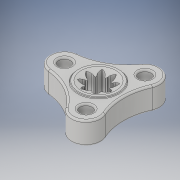
# Autodesk Inventor part: gear sleeve
Saved by Autodesk Inventor 2017 (Build 210142000, 142)
## iProperties
Created: 2020-09-28
Part Number: gear sleeve
Material: Generic
Document SubType Name: Modeling
Designer: Brandt
Density: 1 g/cm^3
Appearance: Default
Author: Brandt
Autodesk Inventor part; units mm, degrees
ref_plane "YZ Plane" through (0, 0, 0) normal (1, 0, 0) x (0, 1, 0)
ref_plane "XZ Plane" through (0, 0, 0) normal (0, 1, 0) x (-1, 0, 0)
ref_plane "XY Plane" through (0, 0, 0) normal (0, 0, 1) x (1, 0, 0)
sketch "Sketch10" plane through (0, 0, 0) normal (0, 1, 0) x (-1, 0, 0)
  circle A0 centre (0, 0) radius 10.9855
  dimension "d120" = 21.971
  constraints: 1 centre point, 1 coincident
  measures "d120" diameter of A0
extrude "Extrusion9" add sketch "Sketch10" along normal blind 5.461
sketch "Sketch12" plane through (0, 0, 0) normal (0, -1, 0) x (-1, 0, 0)
  arc A0 (-1.0187, 1.6285) -> (-1.0516, 1.6075) centre (0, 0) ccw construction
  arc A1 (-1.4637, 1.6634) -> (-1.0516, 1.6075) centre (-1.2254, 1.8732) ccw construction
  line L0 (-1.4637, 1.6634) -> (-1.4758, 1.6771) construction
  arc A2 (-1.4758, 1.6771) -> (-1.5461, 1.7343) centre (-1.6809, 1.4966) ccw construction
  arc A3 (-1.5461, 1.7343) -> (-1.876, 1.8563) centre (-2.085, 0.7843) ccw construction
  arc A4 (-1.876, 1.8563) -> (-2.5953, 1.8563) centre (-2.2357, 0.0114) ccw construction
  arc A5 (-2.5953, 1.8563) -> (-2.6389, 1.7938) centre (0, 0) ccw construction
  arc A6 (-2.6389, 1.7938) -> (-2.3903, 1.1188) centre (-0.7834, 2.0939) ccw construction
  arc A7 (-2.3903, 1.1188) -> (-2.1618, 0.8514) centre (-1.4566, 1.6854) ccw construction
  arc A8 (-2.1618, 0.8514) -> (-2.0838, 0.8052) centre (-1.9853, 1.0601) ccw construction
  line L1 (-2.0838, 0.8052) -> (-2.0668, 0.7986) construction
  arc A9 (-1.8719, 0.4312) -> (-2.0668, 0.7986) centre (-2.1813, 0.5024) ccw construction
  arc A10 (-1.8719, 0.4312) -> (-1.8802, 0.3931) centre (0, 0) ccw construction
  arc A11 (-2.2112, 0.1412) -> (-1.8802, 0.3931) centre (-2.191, 0.4581) ccw construction
  line L2 (-2.2112, 0.1412) -> (-2.2294, 0.1424) construction
  arc A12 (-2.2294, 0.1424) -> (-2.3196, 0.1331) centre (-2.2468, -0.1304) ccw construction
  arc A13 (-2.3196, 0.1331) -> (-2.6391, -0.0139) centre (-2.0289, -0.9197) ccw construction
  arc A14 (-2.6391, -0.0139) -> (-3.1478, -0.5226) centre (-1.5889, -1.5728) ccw construction
  arc A15 (-3.1478, -0.5226) -> (-3.1344, -0.5976) centre (0, 0) ccw construction
  arc A16 (-3.1344, -0.5976) -> (-2.4813, -0.8991) centre (-2.0346, 0.9266) ccw construction
  arc A17 (-2.4813, -0.8991) -> (-2.1306, -0.9266) centre (-2.2217, 0.1618) ccw construction
  arc A18 (-2.1306, -0.9266) -> (-2.0428, -0.9042) centre (-2.1534, -0.6542) ccw construction
  line L3 (-2.0428, -0.9042) -> (-2.0262, -0.8968) construction
  arc A19 (-1.6285, -1.0187) -> (-2.0262, -0.8968) centre (-1.8977, -1.1871) ccw construction
  arc A20 (-1.6285, -1.0187) -> (-1.6075, -1.0516) centre (0, 0) ccw construction
  arc A21 (-1.6634, -1.4637) -> (-1.6075, -1.0516) centre (-1.8732, -1.2254) ccw construction
  line L4 (-1.6634, -1.4637) -> (-1.6771, -1.4758) construction
  arc A22 (-1.6771, -1.4758) -> (-1.7343, -1.5461) centre (-1.4966, -1.6809) ccw construction
  arc A23 (-1.7343, -1.5461) -> (-1.8563, -1.876) centre (-0.7843, -2.085) ccw construction
  arc A24 (-1.8563, -1.876) -> (-1.8563, -2.5953) centre (-0.0114, -2.2357) ccw construction
  arc A25 (-1.8563, -2.5953) -> (-1.7938, -2.6389) centre (0, 0) ccw construction
  arc A26 (-1.7938, -2.6389) -> (-1.1188, -2.3903) centre (-2.0939, -0.7834) ccw construction
  arc A27 (-1.1188, -2.3903) -> (-0.8514, -2.1618) centre (-1.6854, -1.4566) ccw construction
  arc A28 (-0.8514, -2.1618) -> (-0.8052, -2.0838) centre (-1.0601, -1.9853) ccw construction
  line L5 (-0.8052, -2.0838) -> (-0.7986, -2.0668) construction
  arc A29 (-0.4312, -1.8719) -> (-0.7986, -2.0668) centre (-0.5024, -2.1813) ccw construction
  arc A30 (-0.4312, -1.8719) -> (-0.3931, -1.8802) centre (0, 0) ccw construction
  arc A31 (-0.1412, -2.2112) -> (-0.3931, -1.8802) centre (-0.4581, -2.191) ccw construction
  line L6 (-0.1412, -2.2112) -> (-0.1424, -2.2294) construction
  arc A32 (-0.1424, -2.2294) -> (-0.1331, -2.3196) centre (0.1304, -2.2468) ccw construction
  arc A33 (-0.1331, -2.3196) -> (0.0139, -2.6391) centre (0.9197, -2.0289) ccw construction
  arc A34 (0.0139, -2.6391) -> (0.5226, -3.1478) centre (1.5728, -1.5889) ccw construction
  arc A35 (0.5226, -3.1478) -> (0.5976, -3.1344) centre (0, 0) ccw construction
  arc A36 (0.5976, -3.1344) -> (0.8991, -2.4813) centre (-0.9266, -2.0346) ccw construction
  arc A37 (0.8991, -2.4813) -> (0.9266, -2.1306) centre (-0.1618, -2.2217) ccw construction
  arc A38 (0.9266, -2.1306) -> (0.9042, -2.0428) centre (0.6542, -2.1534) ccw construction
  line L7 (0.9042, -2.0428) -> (0.8968, -2.0262) construction
  arc A39 (1.0187, -1.6285) -> (0.8968, -2.0262) centre (1.1871, -1.8977) ccw construction
  arc A40 (1.0187, -1.6285) -> (1.0516, -1.6075) centre (0, 0) ccw construction
  arc A41 (1.4637, -1.6634) -> (1.0516, -1.6075) centre (1.2254, -1.8732) ccw construction
  line L8 (1.4637, -1.6634) -> (1.4758, -1.6771) construction
  arc A42 (1.4758, -1.6771) -> (1.5461, -1.7343) centre (1.6809, -1.4966) ccw construction
  arc A43 (1.5461, -1.7343) -> (1.876, -1.8563) centre (2.085, -0.7843) ccw construction
  arc A44 (1.876, -1.8563) -> (2.5953, -1.8563) centre (2.2357, -0.0114) ccw construction
  arc A45 (2.5953, -1.8563) -> (2.6389, -1.7938) centre (0, 0) ccw construction
  arc A46 (2.6389, -1.7938) -> (2.3903, -1.1188) centre (0.7834, -2.0939) ccw construction
  arc A47 (2.3903, -1.1188) -> (2.1618, -0.8514) centre (1.4566, -1.6854) ccw construction
  arc A48 (2.1618, -0.8514) -> (2.0838, -0.8052) centre (1.9853, -1.0601) ccw construction
  line L9 (2.0838, -0.8052) -> (2.0668, -0.7986) construction
  arc A49 (1.8719, -0.4312) -> (2.0668, -0.7986) centre (2.1813, -0.5024) ccw construction
  arc A50 (1.8719, -0.4312) -> (1.8802, -0.3931) centre (0, 0) ccw construction
  arc A51 (2.2112, -0.1412) -> (1.8802, -0.3931) centre (2.191, -0.4581) ccw construction
  line L10 (2.2112, -0.1412) -> (2.2294, -0.1424) construction
  arc A52 (2.2294, -0.1424) -> (2.3196, -0.1331) centre (2.2468, 0.1304) ccw construction
  arc A53 (2.3196, -0.1331) -> (2.6391, 0.0139) centre (2.0289, 0.9197) ccw construction
  arc A54 (2.6391, 0.0139) -> (3.1478, 0.5226) centre (1.5889, 1.5728) ccw construction
  arc A55 (3.1478, 0.5226) -> (3.1344, 0.5976) centre (0, 0) ccw construction
  arc A56 (3.1344, 0.5976) -> (2.4813, 0.8991) centre (2.0346, -0.9266) ccw construction
  arc A57 (2.4813, 0.8991) -> (2.1306, 0.9266) centre (2.2217, -0.1618) ccw construction
  arc A58 (2.1306, 0.9266) -> (2.0428, 0.9042) centre (2.1534, 0.6542) ccw construction
  line L11 (2.0428, 0.9042) -> (2.0262, 0.8968) construction
  arc A59 (1.6285, 1.0187) -> (2.0262, 0.8968) centre (1.8977, 1.1871) ccw construction
  arc A60 (1.6285, 1.0187) -> (1.6075, 1.0516) centre (0, 0) ccw construction
  arc A61 (1.6634, 1.4637) -> (1.6075, 1.0516) centre (1.8732, 1.2254) ccw construction
  line L12 (1.6634, 1.4637) -> (1.6771, 1.4758) construction
  arc A62 (1.6771, 1.4758) -> (1.7343, 1.5461) centre (1.4966, 1.6809) ccw construction
  arc A63 (1.7343, 1.5461) -> (1.8563, 1.876) centre (0.7843, 2.085) ccw construction
  arc A64 (1.8563, 1.876) -> (1.8563, 2.5953) centre (0.0114, 2.2357) ccw construction
  arc A65 (1.8563, 2.5953) -> (1.7938, 2.6389) centre (0, 0) ccw construction
  arc A66 (1.7938, 2.6389) -> (1.1188, 2.3903) centre (2.0939, 0.7834) ccw construction
  arc A67 (1.1188, 2.3903) -> (0.8514, 2.1618) centre (1.6854, 1.4566) ccw construction
  arc A68 (0.8514, 2.1618) -> (0.8052, 2.0838) centre (1.0601, 1.9853) ccw construction
  line L13 (0.8052, 2.0838) -> (0.7986, 2.0668) construction
  arc A69 (0.4312, 1.8719) -> (0.7986, 2.0668) centre (0.5024, 2.1813) ccw construction
  arc A70 (0.4312, 1.8719) -> (0.3931, 1.8802) centre (0, 0) ccw construction
  arc A71 (0.1412, 2.2112) -> (0.3931, 1.8802) centre (0.4581, 2.191) ccw construction
  line L14 (0.1412, 2.2112) -> (0.1424, 2.2294) construction
  arc A72 (0.1424, 2.2294) -> (0.1331, 2.3196) centre (-0.1304, 2.2468) ccw construction
  arc A73 (0.1331, 2.3196) -> (-0.0139, 2.6391) centre (-0.9197, 2.0289) ccw construction
  arc A74 (-0.0139, 2.6391) -> (-0.5226, 3.1478) centre (-1.5728, 1.5889) ccw construction
  arc A75 (-0.5226, 3.1478) -> (-0.5976, 3.1344) centre (0, 0) ccw construction
  arc A76 (-0.5976, 3.1344) -> (-0.8991, 2.4813) centre (0.9266, 2.0346) ccw construction
  arc A77 (-0.8991, 2.4813) -> (-0.9266, 2.1306) centre (0.1618, 2.2217) ccw construction
  arc A78 (-0.9266, 2.1306) -> (-0.9042, 2.0428) centre (-0.6542, 2.1534) ccw construction
  line L15 (-0.9042, 2.0428) -> (-0.8968, 2.0262) construction
  arc A79 (-1.0187, 1.6285) -> (-0.8968, 2.0262) centre (-1.1871, 1.8977) ccw construction
  circle A80 centre (0, 0) radius 8.0242 construction
  arc A81 (10.9855, 0) -> (10.9855, 0) centre (0, 0) ccw projected
  line L16 (-2.1126, 0.6801) -> (-2.1296, 0.6867)
  arc A82 (-2.2438, 0.7544) -> (-2.1296, 0.6867) centre (-1.9853, 1.0601) ccw
  arc A83 (-2.4989, 1.0529) -> (-2.2438, 0.7544) centre (-1.4566, 1.6854) ccw
  arc A84 (-2.7718, 1.8236) -> (-2.4989, 1.0529) centre (-0.7834, 2.0939) ccw
  arc A85 (-2.6693, 1.9706) -> (-2.7718, 1.8236) centre (0, 0) ccw
  arc A86 (-1.8517, 1.981) -> (-2.6693, 1.9706) centre (-2.2357, 0.0114) ccw
  arc A87 (-1.4834, 1.8448) -> (-1.8517, 1.981) centre (-2.085, 0.7843) ccw
  arc A88 (-1.3804, 1.761) -> (-1.4834, 1.8448) centre (-1.6809, 1.4966) ccw
  line L17 (-1.3804, 1.761) -> (-1.3684, 1.7473)
  arc A89 (-1.3684, 1.7473) -> (-1.1211, 1.7138) centre (-1.2254, 1.8732) ccw
  arc A90 (-1.0861, 1.7361) -> (-1.1211, 1.7138) centre (0, 0) ccw
  arc A91 (-1.0861, 1.7361) -> (-1.0129, 1.9748) centre (-1.1871, 1.8977) ccw
  line L18 (-1.0129, 1.9748) -> (-1.0203, 1.9914)
  arc A92 (-1.0532, 2.12) -> (-1.0203, 1.9914) centre (-0.6542, 2.1534) ccw
  arc A93 (-1.0225, 2.5115) -> (-1.0532, 2.12) centre (0.1618, 2.2217) ccw
  arc A94 (-0.6704, 3.2494) -> (-1.0225, 2.5115) centre (0.9266, 2.0346) ccw
  arc A95 (-0.494, 3.2809) -> (-0.6704, 3.2494) centre (0, 0) ccw
  arc A96 (0.0914, 2.7101) -> (-0.494, 3.2809) centre (-1.5728, 1.5889) ccw
  arc A97 (0.2555, 2.3534) -> (0.0914, 2.7101) centre (-0.9197, 2.0289) ccw
  arc A98 (0.2691, 2.2213) -> (0.2555, 2.3534) centre (-0.1304, 2.2468) ccw
  line L19 (0.2691, 2.2213) -> (0.268, 2.2031)
  arc A99 (0.268, 2.2031) -> (0.4191, 2.0045) centre (0.4581, 2.191) ccw
  arc A100 (0.4597, 1.9956) -> (0.4191, 2.0045) centre (0, 0) ccw
  arc A101 (0.4597, 1.9956) -> (0.6801, 2.1126) centre (0.5024, 2.1813) ccw
  line L20 (0.6801, 2.1126) -> (0.6867, 2.1296)
  arc A102 (0.7544, 2.2438) -> (0.6867, 2.1296) centre (1.0601, 1.9853) ccw
  arc A103 (1.0529, 2.4989) -> (0.7544, 2.2438) centre (1.6854, 1.4566) ccw
  arc A104 (1.8236, 2.7718) -> (1.0529, 2.4989) centre (2.0939, 0.7834) ccw
  arc A105 (1.9706, 2.6693) -> (1.8236, 2.7718) centre (0, 0) ccw
  arc A106 (1.981, 1.8517) -> (1.9706, 2.6693) centre (0.0114, 2.2357) ccw
  arc A107 (1.8448, 1.4834) -> (1.981, 1.8517) centre (0.7843, 2.085) ccw
  arc A108 (1.761, 1.3804) -> (1.8448, 1.4834) centre (1.4966, 1.6809) ccw
  line L21 (1.761, 1.3804) -> (1.7473, 1.3684)
  arc A109 (1.7473, 1.3684) -> (1.7138, 1.1211) centre (1.8732, 1.2254) ccw
  arc A110 (1.7361, 1.0861) -> (1.7138, 1.1211) centre (0, 0) ccw
  arc A111 (1.7361, 1.0861) -> (1.9748, 1.0129) centre (1.8977, 1.1871) ccw
  line L22 (1.9748, 1.0129) -> (1.9914, 1.0203)
  arc A112 (2.12, 1.0532) -> (1.9914, 1.0203) centre (2.1534, 0.6542) ccw
  arc A113 (2.5115, 1.0225) -> (2.12, 1.0532) centre (2.2217, -0.1618) ccw
  arc A114 (3.2494, 0.6704) -> (2.5115, 1.0225) centre (2.0346, -0.9266) ccw
  arc A115 (3.2809, 0.494) -> (3.2494, 0.6704) centre (0, 0) ccw
  arc A116 (2.7101, -0.0914) -> (3.2809, 0.494) centre (1.5889, 1.5728) ccw
  arc A117 (2.3534, -0.2555) -> (2.7101, -0.0914) centre (2.0289, 0.9197) ccw
  arc A118 (2.2213, -0.2691) -> (2.3534, -0.2555) centre (2.2468, 0.1304) ccw
  line L23 (2.2213, -0.2691) -> (2.2031, -0.268)
  arc A119 (2.2031, -0.268) -> (2.0045, -0.4191) centre (2.191, -0.4581) ccw
  arc A120 (1.9956, -0.4597) -> (2.0045, -0.4191) centre (0, 0) ccw
  arc A121 (1.9956, -0.4597) -> (2.1126, -0.6801) centre (2.1813, -0.5024) ccw
  line L24 (2.1126, -0.6801) -> (2.1296, -0.6867)
  arc A122 (2.2438, -0.7544) -> (2.1296, -0.6867) centre (1.9853, -1.0601) ccw
  arc A123 (2.4989, -1.0529) -> (2.2438, -0.7544) centre (1.4566, -1.6854) ccw
  arc A124 (2.7718, -1.8236) -> (2.4989, -1.0529) centre (0.7834, -2.0939) ccw
  arc A125 (2.6693, -1.9706) -> (2.7718, -1.8236) centre (0, 0) ccw
  arc A126 (1.8517, -1.981) -> (2.6693, -1.9706) centre (2.2357, -0.0114) ccw
  arc A127 (1.4834, -1.8448) -> (1.8517, -1.981) centre (2.085, -0.7843) ccw
  arc A128 (1.3804, -1.761) -> (1.4834, -1.8448) centre (1.6809, -1.4966) ccw
  line L25 (1.3804, -1.761) -> (1.3684, -1.7473)
  arc A129 (1.3684, -1.7473) -> (1.1211, -1.7138) centre (1.2254, -1.8732) ccw
  arc A130 (1.0861, -1.7361) -> (1.1211, -1.7138) centre (0, 0) ccw
  arc A131 (1.0861, -1.7361) -> (1.0129, -1.9748) centre (1.1871, -1.8977) ccw
  line L26 (1.0129, -1.9748) -> (1.0203, -1.9914)
  arc A132 (1.0532, -2.12) -> (1.0203, -1.9914) centre (0.6542, -2.1534) ccw
  arc A133 (1.0225, -2.5115) -> (1.0532, -2.12) centre (-0.1618, -2.2217) ccw
  arc A134 (0.6704, -3.2494) -> (1.0225, -2.5115) centre (-0.9266, -2.0346) ccw
  arc A135 (0.494, -3.2809) -> (0.6704, -3.2494) centre (0, 0) ccw
  arc A136 (-0.0914, -2.7101) -> (0.494, -3.2809) centre (1.5728, -1.5889) ccw
  arc A137 (-0.2555, -2.3534) -> (-0.0914, -2.7101) centre (0.9197, -2.0289) ccw
  arc A138 (-0.2691, -2.2213) -> (-0.2555, -2.3534) centre (0.1304, -2.2468) ccw
  line L27 (-0.2691, -2.2213) -> (-0.268, -2.2031)
  arc A139 (-0.268, -2.2031) -> (-0.4191, -2.0045) centre (-0.4581, -2.191) ccw
  arc A140 (-0.4597, -1.9956) -> (-0.4191, -2.0045) centre (0, 0) ccw
  arc A141 (-0.4597, -1.9956) -> (-0.6801, -2.1126) centre (-0.5024, -2.1813) ccw
  line L28 (-0.6801, -2.1126) -> (-0.6867, -2.1296)
  arc A142 (-0.7544, -2.2438) -> (-0.6867, -2.1296) centre (-1.0601, -1.9853) ccw
  arc A143 (-1.0529, -2.4989) -> (-0.7544, -2.2438) centre (-1.6854, -1.4566) ccw
  arc A144 (-1.8236, -2.7718) -> (-1.0529, -2.4989) centre (-2.0939, -0.7834) ccw
  arc A145 (-1.9706, -2.6693) -> (-1.8236, -2.7718) centre (0, 0) ccw
  arc A146 (-1.981, -1.8517) -> (-1.9706, -2.6693) centre (-0.0114, -2.2357) ccw
  arc A147 (-1.8448, -1.4834) -> (-1.981, -1.8517) centre (-0.7843, -2.085) ccw
  arc A148 (-1.761, -1.3804) -> (-1.8448, -1.4834) centre (-1.4966, -1.6809) ccw
  line L29 (-1.761, -1.3804) -> (-1.7473, -1.3684)
  arc A149 (-1.7473, -1.3684) -> (-1.7138, -1.1211) centre (-1.8732, -1.2254) ccw
  arc A150 (-1.7361, -1.0861) -> (-1.7138, -1.1211) centre (0, 0) ccw
  arc A151 (-1.7361, -1.0861) -> (-1.9748, -1.0129) centre (-1.8977, -1.1871) ccw
  line L30 (-1.9748, -1.0129) -> (-1.9914, -1.0203)
  arc A152 (-2.12, -1.0532) -> (-1.9914, -1.0203) centre (-2.1534, -0.6542) ccw
  arc A153 (-2.5115, -1.0225) -> (-2.12, -1.0532) centre (-2.2217, 0.1618) ccw
  arc A154 (-3.2494, -0.6704) -> (-2.5115, -1.0225) centre (-2.0346, 0.9266) ccw
  arc A155 (-3.2809, -0.494) -> (-3.2494, -0.6704) centre (0, 0) ccw
  arc A156 (-2.7101, 0.0914) -> (-3.2809, -0.494) centre (-1.5889, -1.5728) ccw
  arc A157 (-2.3534, 0.2555) -> (-2.7101, 0.0914) centre (-2.0289, -0.9197) ccw
  arc A158 (-2.2213, 0.2691) -> (-2.3534, 0.2555) centre (-2.2468, -0.1304) ccw
  line L31 (-2.2213, 0.2691) -> (-2.2031, 0.268)
  arc A159 (-2.2031, 0.268) -> (-2.0045, 0.4191) centre (-2.191, 0.4581) ccw
  arc A160 (-1.9956, 0.4597) -> (-2.0045, 0.4191) centre (0, 0) ccw
  arc A161 (-1.9956, 0.4597) -> (-2.1126, 0.6801) centre (-2.1813, 0.5024) ccw
  point P0 (0, 0)
  point P1 (-2.4121, -4.6897)
  point P2 (-2.3763, -4.708)
  dimension "d100" = 0.127
  constraints: 320 point on circle, 161 centre point, 64 end point, 97 other
  measures "d100" radial gap between concentric circles of A9 A161
extrude "Extrusion11" cut sketch "Sketch12" against normal through all contours L16 A82 A83 A84 A85 A86 A87 A88 L17 A89 A90 A91 L18 A92 A93 A94 A95 A96 A97 A98 L19 A99 A100 A101 L20 A102 A103 A104 A105 A106 A107 A108 L21 A109 A110 A111 L22 A112 A113 A114 A115 A116 A117 A118 L23 A119 A120 A121 L24 A122 A123 A124 A125 A126 A127 A128 L25 A129 A130 A131 L26 A132 A133 A134 A135 A136 A137 A138 L27 A139 A140 A141 L28 A142 A143 A144 A145 A146 A147 A148 L29 A149 A150 A151 L30 A152 A153 A154 A155 A156 A157 A158 L31 A159 A160 A161
sketch "Sketch13" plane through (0, 0, 0) normal (1, 0, 0) x (0, 1, 0)
  line L0 (5.461, 0) -> (3.8828, 0)
  line L1 (3.8828, 0) -> (5.461, -3.81)
  line L2 (5.461, -3.81) -> (5.461, 0)
  line L3 (-1.0922, 0) -> (6.5532, 0) projected
  line L4 (5.461, -10.9855) -> (5.461, 10.9855) projected
  point P0 (0, 0)
  point P1 (5.461, 1.9956)
  dimension "d106" = 22.5
  dimension "d119" = 3.81
  constraints: 6 end point, 2 point on line, 1 horizontal, 1 vertical
  measures "d106" angle of L1 L2
  measures "d119" distance from line of L3 L1.end
revolve "Revolution1" cut sketch "Sketch13" angle 360 about axis through (0, -10, 0) along (0, 1, 0)
sketch "Sketch14" plane through (0, 5.461, 0) normal (0, 1, 0) x (1, 0, 0)
  circle A0 centre (0, 0) radius 4.445
  circle A1 centre (0, 0) radius 12.7
  dimension "d110" = 8.89
  dimension "d111" = 25.4
  constraints: 2 centre point, 2 coincident
  measures "d110" diameter of A0
  measures "d111" diameter of A1
extrude "Extrusion12" cut sketch "Sketch14" against normal blind 0.254
sketch "Sketch15" plane through (0, 0, 0) normal (0, -1, 0) x (1, 0, 0)
  circle A0 centre (0, 0) radius 4.445
  circle A1 centre (0, 0) radius 12.7
  dimension "d114" = 8.89
  dimension "d115" = 25.4
  constraints: 2 centre point, 2 coincident
  measures "d114" diameter of A0
  measures "d115" diameter of A1
extrude "Extrusion13" cut sketch "Sketch15" against normal blind 0.254
fillet "Fillet6" radius 0.127 4 edges at (-4.445, 0.254, 0) (-4.445, 0, 0) (-4.445, 5.207, 0) (-4.445, 5.461, 0)
sketch "Sketch16" plane through (0, 5.207, 0) normal (0, 1, 0) x (1, 0, 0)
  circle A0 centre (0, 0) radius 7.4549 construction
  circle A1 centre (-7.4549, 0) radius 1.3335
  circle A2 centre (3.7274, -6.4561) radius 1.3335
  circle A3 centre (3.7275, 6.4561) radius 1.3335
  line L0 (-7.4549, 0) -> (0, 0) construction
  dimension "d121" = 14.9098
  dimension "d124" = 360
  dimension "d126" = 2.667
  constraints: 3 centre point, 2 end point, 1 coincident, 1 horizontal, 1 horizontal alignment, 9 other
  measures "d126" diameter of A1
extrude "Extrusion14" cut sketch "Sketch16" against normal through all
sketch "Sketch17" plane through (0, 5.207, 0) normal (0, 1, 0) x (1, 0, 0)
  circle A0 centre (-7.4549, 0) radius 1.3335 projected
  circle A1 centre (3.7275, 6.4561) radius 1.3335 projected
  circle A2 centre (3.7274, -6.4561) radius 1.3335 projected
  circle A3 centre (-7.4549, 0) radius 1.3335 projected
  arc A4 (-7.787, 3.1576) -> (-7.787, -3.1576) centre (-7.4549, 0) ccw
  arc A5 (6.628, 5.1649) -> (1.1589, 8.3225) centre (3.7275, 6.4561) ccw
  arc A6 (1.1589, -8.3225) -> (6.628, -5.1649) centre (3.7274, -6.4561) ccw
  arc A7 (-7.787, 3.1576) -> (1.1589, 8.3225) centre (-9.1152, 15.7879) ccw
  arc A8 (6.628, 5.1649) -> (6.628, -5.1649) centre (18.2303, 0) ccw
  arc A9 (1.1589, -8.3225) -> (-7.787, -3.1576) centre (-9.1152, -15.7879) ccw
  circle A10 centre (0, 0) radius 12.7
  dimension "d129" = 6.35
  dimension "d130" = 6.35
  dimension "d131" = 6.35
  dimension "d132" = 12.7
  dimension "d133" = 12.7
  dimension "d134" = 12.7
  dimension "d135" = 25.4
  constraints: 12 point on circle, 7 centre point, 6 tangent, 4 coincident
  measures "d129" diameter of A4
  measures "d130" diameter of A5
  measures "d131" diameter of A6
  measures "d132" radius of A7
  measures "d133" radius of A8
  measures "d134" radius of A9
  measures "d135" diameter of A10
extrude "Extrusion15" cut sketch "Sketch17" against normal through all contours A10
fillet "Fillet7" radius 0.381 18 edges at (5.315, 5.207, -9.2058) (-2.7652, 5.207, -4.7894) (-10.6299, 5.207, 0) (-2.7652, 5.207, 4.7894) (5.3149, 5.207, 9.2058) (5.5303, 5.207, 0) (5.3149, 0.254, 9.2058) (-2.7652, 0.254, 4.7894) (-10.6299, 0.254, 0) (-2.7652, 0.254, -4.7894) (5.315, 0.254, -9.2058) (5.5303, 0.254, 0) (2.3939, 5.207, 6.4561) (-8.7884, 5.207, 0) (2.394, 5.207, -6.4561) (2.3939, 0.254, 6.4561) (2.394, 0.254, -6.4561) (-8.7884, 0.254, 0)
equation "\"Bottom_Ratio\" = 0.333333"
body "Solid1"
